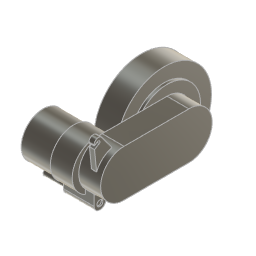
robotCad (Autodesk Fusion 360 archive; units mm, degrees)
design "silnikLewyDok"
Autodesk Fusion 360 part; units mm, degrees
sketch "Szkic1" plane through (0, 0, 0) normal (1, 0, 0) x (0, 1, 0)
  circle A0 centre (0, 0) radius 32.5
  dimension "d1" = 65
  constraint coincident A0.centre origin
  measures "d1" diameter of A0
extrude "Wyciągnięcie proste1" add sketch "Szkic1" along normal blind 15.5 makes body 1
sketch "Szkic2" plane through (15.5, 0, 0) normal (1, 0, 0) x (0, 1, 0)
  circle A0 centre (0, 0) radius 32.5
  circle A1 centre (0, 0) radius 23
  dimension "d4" = 46
  constraint coincident A0.centre A1.centre
  measures "d4" diameter of A1
extrude "Wyciągnięcie proste2" add sketch "Szkic2" along normal blind 2 contours A1 bodies 1
sketch "Szkic3" plane through (17.5, 0, 0) normal (1, 0, 0) x (0, 1, 0)
  circle A0 centre (0, 0) radius 23
  circle A1 centre (0, 0) radius 16
  circle A2 centre (-44.5, 0) radius 16
  line L0 (-44.5, 16) -> (0, 16)
  line L1 (-44.5, -16) -> (0, -16)
  dimension "d7" = 32
  dimension "d8" = 32
  dimension "d9" = 44.5
  constraint concentric A0 A1
  constraint tangent A2 L0
  constraint tangent A1 L0
  constraint coincident A2 L0.start
  constraint tangent A1 L1
  constraint coincident A2 L1.start
  constraint tangent A2 L1
  constraint coincident A1 L1.end
  constraint coincident A1 L0.end
  measures "d7" diameter of A1
  measures "d8" diameter of A2
  measures "d9" distance of A0.centre A2.centre
extrude "Wyciągnięcie proste3" add sketch "Szkic3" along normal blind 15 contours A0 A1 L0 L1 | A0 A2 L0 L1 | A2 | A1 picked at (-15.8747, 13.172) bodies 1
sketch "Szkic4" plane through (17.5, 0, 0) normal (-1, 0, 0) x (0, -1, 0)
  arc A0 (16.5227, -16) -> (16.5227, 16) centre (0, 0) ccw
  line L0 (16.5227, -16) -> (44.5, -16)
  arc A1 (44.5, -16) -> (44.5, 16) centre (44.5, 0) ccw
  line L1 (44.5, 16) -> (16.5227, 16)
  circle A2 centre (49, 0) radius 16
  arc A3 (0, 16) -> (0, -16) centre (0, 0) ccw
  circle A4 centre (49, 0) radius 15
  dimension "d12" = 32
  dimension "d13" = 49
  dimension "d14" = 30
  constraint concentric A2 A4
  measures "d12" diameter of A2
  measures "d13" distance of A2.centre A0.centre
  measures "d14" diameter of A4
extrude "Wyciągnięcie proste4" add sketch "Szkic4" along normal blind 15 contours A1 A2 A4 | A1 A2 A4 bodies 1
sketch "Szkic5" plane through (17.5, 0, 0) normal (-1, 0, 0) x (0, -1, 0)
  arc A0 (50.1944, 14.9524) -> (50.1944, -14.9524) centre (49, 0) ccw
  arc A1 (50.1944, -14.9524) -> (50.1944, 14.9524) centre (44.5, 0) ccw
  circle A2 centre (49, 0) radius 15
  circle A3 centre (49, 0) radius 15
  constraint concentric A0 A2
  constraint tangent A2 A3
extrude "Wyciągnięcie proste5" add sketch "Szkic5" along normal blind 36 bodies 1
ref_plane "Płaszczyzna konstrukcyjna1" through (23.5, -22.25, 0) normal (1, 0, 0) x (0, 1, 0)
sketch "Szkic6" plane through (23.5, -22.25, 0) normal (1, 0, 0) x (0, 1, 0)
  circle A0 centre (-29.75, -18.5) radius 2
  circle A1 centre (-29.75, -18.5) radius 4
  arc A2 (-22.25, 16) -> (-22.25, -16) centre (-22.25, 0) ccw
  arc A3 (22.25, -16) -> (22.25, 16) centre (22.25, 0) ccw
  point P0 (-16, -22.5)
  dimension "d20" = 4
  dimension "d21" = 8
  dimension "d22" = 22.5
  dimension "d23" = 4
  dimension "d24" = 52
  constraint concentric A0 A1
  measures "d20" diameter of A0
  measures "d21" diameter of A1
  measures "d22" vertical distance of P0 A2.centre
  measures "d23" vertical distance of A0.centre P0
  measures "d24" horizontal distance of A0.centre A3.centre
extrude "Wyciągnięcie proste6" add sketch "Szkic6" against normal blind 21 separate body contours A1 A2 picked at (-33.0386, -18.0016) makes body 2
sketch "Szkic8" plane through (23.5, 0, 0) normal (1, 0, 0) x (0, 1, 0)
  circle A0 centre (-52, -18.5) radius 2
  circle A1 centre (-52, -18.5) radius 2
  arc A2 (-50.962, -14.637) -> (-50.0549, -15.0048) centre (-52, -18.5) ccw
  arc A3 (-50.962, -14.637) -> (-50.0549, -15.0048) centre (-44.5, 0) ccw
  constraint concentric A0 A1
extrude "Wyciągnięcie proste7" add sketch "Szkic8" along normal blind -37 and the other way blind 1 contours A0 A1 bodies 2
sketch "Szkic9" plane through (23.5, 0, 0) normal (1, 0, 0) x (0, 1, 0)
  line L0 (-48.4419, -20.3275) -> (-46.1741, -15.9122)
  arc A0 (-44.5, 16) -> (-44.5, -16) centre (-44.5, 0) ccw
  line L1 (-56, -18.5) -> (-56, -11.1243)
  line L2 (-46.1741, -15.9122) -> (-56, -11.1243)
  arc A1 (-50.962, -14.637) -> (-50.0549, -15.0048) centre (-52, -18.5) ccw
  arc A2 (-50.962, -14.637) -> (-50.0549, -15.0048) centre (-44.5, 0) ccw
  circle A3 centre (-52, -18.5) radius 2
  constraint tangent L0 A1
  constraint coincident L0.start A1
  constraint coincident L1.start A1
  constraint coincident A0 L1.end
  constraint vertical L1
  constraint coincident A0 L0.end
extrude "Wyciągnięcie proste8" add sketch "Szkic9" against normal up to surface (21 mm away) contours L0 A0 A1 | A0 L2 A2 | A0 L1 A1 bodies 1 2
ref_plane "Płaszczyzna konstrukcyjna2" through (28.5, -22.25, 0) normal (1, 0, 0) x (0, 1, 0)
sketch "Szkic10" plane through (28.5, -22.25, 0) normal (1, 0, 0) x (0, 1, 0)
  circle A0 centre (-35.75, 23) radius 3
  line L0 (-38.75, -16) -> (-38.75, 26) construction
  line L1 (-38.75, 26) -> (-16.3036, 26) construction
  line L2 (-22.25, -16) -> (22.25, -16)
  arc A1 (-24.5, 15.841) -> (-33.75, -14.3875) centre (-26.75, 0) ccw
  arc A2 (-22.25, 16) -> (-22.25, -16) centre (-22.25, 0) ccw
  line L3 (-38.75, 23) -> (-37.0399, 6.104)
  line L4 (-33.5801, 25.0716) -> (-26.5025, 15.4245)
  dimension "d35" = 6
  dimension "d36" = 42
  dimension "d37" = 16.5
  constraint vertical L0
  constraint perpendicular L0 L1
  constraint tangent A0 L1
  constraint coincident L0.start L2
  constraint tangent A0 L0
  constraint coincident A0 L3.start
  constraint coincident A2 L3.end
  constraint coincident A0 L4.start
  constraint coincident A2 L4.end
  measures "d35" diameter of A0
  measures "d36" distance of L0.start L0.end
  measures "d37" distance of L0 A2.centre
extrude "Wyciągnięcie proste9" add sketch "Szkic10" against normal blind 3.5 contours A0 L3 L4 | A0 A1 L3 L4 | A1 A2 L3 L4 bodies 1
sketch "Szkic11" plane through (28.5, 0, 0) normal (1, 0, 0) x (0, 1, 0)
  line L0 (-61, 23) -> (-59.2899, 6.104)
  arc A0 (-48.7525, 15.4245) -> (-59.2899, 6.104) centre (-44.5, 0) ccw
  line L1 (-48.7525, 15.4245) -> (-55.8301, 25.0716)
  arc A1 (-55.8301, 25.0716) -> (-61, 23) centre (-58, 23) ccw
  circle A2 centre (-58, 23) radius 1
  line L2 (-57.4724, 22.1505) -> (-60.7105, 20.1395)
  line L3 (-58.4492, 23.8935) -> (-61.2557, 22.1505)
  dimension "d40" = 2
  constraint concentric A1 A2
  constraint coincident A2 L2.start
  constraint coincident L0 L2.end
  constraint tangent A2 L2
  constraint coincident A2 L3.start
  constraint parallel L2 L3
  measures "d40" distance of A1 A2
extrude "Wyciągnięcie proste10" cut sketch "Szkic11" against normal blind 10 contours A2 | L0 A2 L2 L3 bodies 1
equation "d9 = 75.5 mm - 31 mm"
equation "d13 = 81 mm - 32 mm"
equation "d22 = 38.5 mm - 16 mm"
equation "d24 = 56 mm - 4 mm"

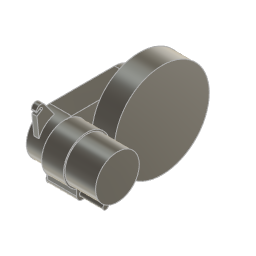
design "silnikPrawyDok"
Autodesk Fusion 360 part; units mm, degrees
sketch "Szkic1" plane through (0, 0, 0) normal (1, 0, 0) x (0, 1, 0)
  circle A0 centre (0, 0) radius 32.5
  dimension "d1" = 65
  constraint coincident A0.centre origin
  measures "d1" diameter of A0
extrude "Wyciągnięcie proste1" add sketch "Szkic1" along normal blind 15.5 makes body 1
sketch "Szkic2" plane through (0, 0, 0) normal (1, 0, 0) x (0, 1, 0)
  circle A0 centre (0, 0) radius 32.5
  circle A1 centre (0, 0) radius 23
  circle A2 centre (0, 0) radius 32.5
  dimension "d4" = 46
  constraint coincident A0.centre A1.centre
  measures "d4" diameter of A1
extrude "Wyciągnięcie proste2" add sketch "Szkic2" against normal blind 2 contours A1 bodies 1
sketch "Szkic3" plane through (-2, 0, 0) normal (-1, 0, 0) x (0, 1, 0)
  circle A0 centre (0, 0) radius 23
  circle A1 centre (0, 0) radius 16
  circle A2 centre (-44.5, 0) radius 16
  line L0 (-44.5, 16) -> (0, 16)
  line L1 (-44.5, -16) -> (0, -16)
  dimension "d7" = 32
  dimension "d8" = 32
  dimension "d9" = 44.5
  constraint concentric A0 A1
  constraint tangent A2 L0
  constraint tangent A1 L0
  constraint coincident A2 L0.start
  constraint tangent A1 L1
  constraint coincident A2 L1.start
  constraint tangent A2 L1
  constraint coincident A1 L1.end
  constraint coincident A1 L0.end
  measures "d7" diameter of A1
  measures "d8" diameter of A2
  measures "d9" distance of A0.centre A2.centre
extrude "Wyciągnięcie proste3" add sketch "Szkic3" along normal blind 15 contours A0 A1 L0 L1 | A0 A2 L0 L1 | A2 | A1 picked at (-15.8747, 13.172) bodies 1
sketch "Szkic4" plane through (-2, 0, 0) normal (1, 0, 0) x (0, -1, 0)
  arc A0 (16.5227, -16) -> (16.5227, 16) centre (0, 0) ccw
  line L0 (16.5227, -16) -> (44.5, -16)
  arc A1 (44.5, -16) -> (44.5, 16) centre (44.5, 0) ccw
  line L1 (44.5, 16) -> (16.5227, 16)
  circle A2 centre (49, 0) radius 16
  arc A3 (0, 16) -> (0, -16) centre (0, 0) ccw
  circle A4 centre (49, 0) radius 15
  dimension "d12" = 32
  dimension "d13" = 49
  dimension "d14" = 30
  constraint concentric A2 A4
  measures "d12" diameter of A2
  measures "d13" distance of A2.centre A0.centre
  measures "d14" diameter of A4
extrude "Wyciągnięcie proste4" add sketch "Szkic4" along normal blind 15 contours A1 A2 A4 | A1 A2 A4 bodies 1
sketch "Szkic5" plane through (-2, 0, 0) normal (1, 0, 0) x (0, -1, 0)
  arc A0 (50.1944, 14.9524) -> (50.1944, -14.9524) centre (49, 0) ccw
  arc A1 (50.1944, -14.9524) -> (50.1944, 14.9524) centre (44.5, 0) ccw
  circle A2 centre (49, 0) radius 15
  circle A3 centre (49, 0) radius 15
  constraint concentric A0 A2
  constraint tangent A2 A3
extrude "Wyciągnięcie proste5" add sketch "Szkic5" along normal blind 36 bodies 1
ref_plane "Płaszczyzna konstrukcyjna1" through (-8, -22.25, 0) normal (-1, 0, 0) x (0, 1, 0)
sketch "Szkic6" plane through (-8, -22.25, 0) normal (-1, 0, 0) x (0, 1, 0)
  circle A0 centre (-29.75, -18.5) radius 2
  circle A1 centre (-29.75, -18.5) radius 4
  arc A2 (-22.25, 16) -> (-22.25, -16) centre (-22.25, 0) ccw
  arc A3 (22.25, -16) -> (22.25, 16) centre (22.25, 0) ccw
  line L0 (42.25, 0) -> (24.75, 0)
  circle A4 centre (-29.75, 18.5) radius 2
  circle A5 centre (-29.75, 18.5) radius 4
  point P0 (-16, -22.5)
  dimension "d20" = 4
  dimension "d21" = 8
  dimension "d22" = 22.5
  dimension "d23" = 4
  dimension "d24" = 52
  constraint concentric A0 A1
  constraint symmetric A0 L0 A4
  constraint symmetric A1 L0 A5
  measures "d20" diameter of A0
  measures "d21" diameter of A1
  measures "d22" vertical distance of P0 A2.centre
  measures "d23" vertical distance of A0.centre P0
  measures "d24" horizontal distance of A0.centre A3.centre
extrude "Wyciągnięcie proste6" add sketch "Szkic6" against normal blind 21 separate body contours A2 A5 picked at (-33.0386, 18.0016) makes body 2
sketch "Szkic8" plane through (-8, 0, 0) normal (-1, 0, 0) x (0, 1, 0)
  circle A0 centre (-52, -18.5) radius 2
  arc A1 (-50.0549, 15.0048) -> (-50.962, 14.637) centre (-44.5, 0) ccw
  circle A2 centre (-52, 18.5) radius 2
  arc A3 (-50.0549, 15.0048) -> (-50.962, 14.637) centre (-52, 18.5) ccw
extrude "Wyciągnięcie proste7" add sketch "Szkic8" along normal blind -37 and the other way blind 1 contours A2 bodies 2
sketch "Szkic9" plane through (-7, 0, 0) normal (-1, 0, 0) x (0, 1, 0)
  line L0 (-48.4419, -20.3275) -> (-46.1741, -15.9122)
  arc A0 (-44.5, 16) -> (-44.5, -16) centre (-44.5, 0) ccw
  line L1 (-56, -18.5) -> (-56, -11.1243)
  line L2 (-46.1741, -15.9122) -> (-56, -11.1243)
  arc A1 (-50.0549, 15.0048) -> (-50.962, 14.637) centre (-44.5, 0) ccw
  circle A2 centre (-52, 18.5) radius 2
  circle A3 centre (-52, 18.5) radius 2
  arc A4 (-50.0549, 15.0048) -> (-50.962, 14.637) centre (-52, 18.5) ccw
  line L3 (20, 0) -> (2.5, 0)
  line L4 (-56, 18.5) -> (-56, 11.1243)
  line L5 (-46.1741, 15.9122) -> (-56, 11.1243)
  line L6 (-48.4419, 20.3275) -> (-46.1741, 15.9122)
  point P0 (-44.5, 16)
  constraint coincident A0 L1.end
  constraint vertical L1
  constraint coincident A0 L0.end
  constraint symmetric L0.start L3 L6.start
  constraint symmetric A0.end L3 P0
  constraint symmetric L0.end L3 L5.start
  constraint symmetric L1.start L3 L4.start
  constraint symmetric L1.end L3 L4.end
extrude "Wyciągnięcie proste8" add sketch "Szkic9" against normal up to surface (20 mm away) contours A0 A1 L5 | A0 A4 L6 | A0 A4 L4 bodies 1 2
ref_plane "Płaszczyzna konstrukcyjna2" through (-13, -22.25, 0) normal (-1, 0, 0) x (0, 1, 0)
sketch "Szkic10" plane through (-13, -22.25, 0) normal (-1, 0, 0) x (0, 1, 0)
  circle A0 centre (-35.75, 23) radius 3
  line L0 (-38.75, -16) -> (-38.75, 26) construction
  line L1 (-38.75, 26) -> (-16.3036, 26) construction
  line L2 (-22.25, -16) -> (22.25, -16)
  arc A1 (-33.75, 14.3875) -> (-24.5, -15.841) centre (-26.75, 0) ccw
  arc A2 (-22.25, 16) -> (-22.25, -16) centre (-22.25, 0) ccw
  line L3 (-38.75, 23) -> (-37.0399, 6.104)
  line L4 (-33.5801, 25.0716) -> (-26.5025, 15.4245)
  line L5 (42.25, 0) -> (24.75, 0)
  line L6 (-33.5801, -25.0716) -> (-26.5025, -15.4245)
  circle A3 centre (-35.75, -23) radius 3
  line L7 (-38.75, -23) -> (-37.0399, -6.104)
  point P0 (-22.25, -16)
  point P1 (-33.75, -14.3875)
  point P2 (-38.75, -26)
  dimension "d35" = 6
  dimension "d36" = 42
  dimension "d37" = 16.5
  constraint vertical L0
  constraint perpendicular L0 L1
  constraint tangent A0 L1
  constraint coincident L0.start L2
  constraint tangent A0 L0
  constraint coincident A0 L3.start
  constraint coincident A2 L3.end
  constraint coincident A0 L4.start
  constraint coincident A2 L4.end
  constraint symmetric A0 L5 A3
  constraint symmetric L0.end L5 P2
  constraint symmetric A1.start L5 P1
  constraint symmetric A2.start L5 P0
  constraint symmetric L3.start L5 L7.start
  constraint symmetric L3.end L5 L7.end
  constraint symmetric L4.start L5 L6.start
  constraint symmetric L4.end L5 L6.end
  measures "d35" diameter of A0
  measures "d36" distance of L0.start L0.end
  measures "d37" distance of L0 A2.centre
extrude "Wyciągnięcie proste9" add sketch "Szkic10" against normal blind 3.5 contours A1 A2 L6 L7 | A1 L6 A3 L7 | L6 A3 L7 bodies 1
sketch "Szkic11" plane through (-13, 0, 0) normal (-1, 0, 0) x (0, 1, 0)
  arc A0 (-59.2899, -6.104) -> (-48.7525, -15.4245) centre (-44.5, 0) ccw
  circle A1 centre (-58, 23) radius 1
  line L0 (-57.4724, 22.1505) -> (-60.7105, 20.1395)
  line L1 (-58.4492, 23.8935) -> (-61.2557, 22.1505)
  line L2 (-55.8301, -25.0716) -> (-48.7525, -15.4245)
  line L3 (-59.2899, -6.104) -> (-61, -23)
  arc A2 (-61, -23) -> (-55.8301, -25.0716) centre (-58, -23) ccw
  line L4 (20, 0) -> (2.5, 0)
  circle A3 centre (-58, -23) radius 1
  line L5 (-57.4724, -22.1505) -> (-60.7105, -20.1395)
  line L6 (-58.4492, -23.8935) -> (-61.2557, -22.1505)
  constraint coincident A1 L0.start
  constraint tangent A1 L0
  constraint coincident A1 L1.start
  constraint parallel L0 L1
  constraint symmetric A1 L4 A3
  constraint symmetric L0.start L4 L5.start
  constraint symmetric L0.end L4 L5.end
  constraint symmetric L1.start L4 L6.start
  constraint symmetric L1.end L4 L6.end
extrude "Wyciągnięcie proste10" cut sketch "Szkic11" against normal blind 10 contours L3 A3 L5 L6 | A3 L6 | A1 L1 picked at (-57.7688, -22.7789) picked at (-57.8523, 23.2601) bodies 1
equation "d9 = 75.5 mm - 31 mm"
equation "d13 = 81 mm - 32 mm"
equation "d22 = 38.5 mm - 16 mm"
equation "d24 = 56 mm - 4 mm"

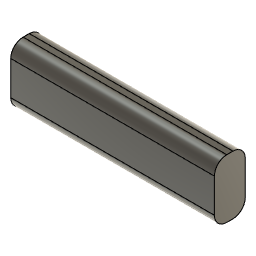
design "bat4s1p_dluga"
Autodesk Fusion 360 part; units mm, degrees
sketch "Szkic1" plane through (0, 0, 0) normal (1, 0, 0) x (0, 1, 0)
  line L0 (8, 25) -> (12, 25)
  line L1 (20, 17) -> (20, -5)
  line L2 (12, -13) -> (8, -13)
  line L3 (0, -5) -> (0, 17)
  arc A0 (8, 25) -> (0, 17) centre (8, 17) ccw
  arc A1 (20, 17) -> (12, 25) centre (12, 17) ccw
  arc A2 (12, -13) -> (20, -5) centre (12, -5) ccw
  arc A3 (0, -5) -> (8, -13) centre (8, -5) ccw
  point P0 (0, 25)
  point P1 (20, 25)
  point P2 (20, -13)
  dimension "d1" = 20
  dimension "d2" = 38
  dimension "d3" = 8
  dimension "d4" = 8
  constraint horizontal L0
  constraint vertical L1
  constraint horizontal L2
  constraint vertical L3
  constraint coincident P0 L0
  constraint coincident P0 L3
  constraint tangent L0 A0
  constraint tangent L3 A0
  constraint coincident P1 L0
  constraint coincident P1 L1
  constraint tangent L0 A1
  constraint tangent L1 A1
  constraint coincident P2 L1
  constraint coincident P2 L2
  constraint tangent L1 A2
  constraint tangent L2 A2
  constraint equal A1 A2
  constraint tangent L2 A3
  constraint tangent L3 A3
  constraint equal A1 A3
  measures "d1" distance of P0 P1
  measures "d2" distance of P1 P2
  measures "d3" radius of A0
  measures "d4" radius of A1
extrude "Wyciągnięcie proste1" add sketch "Szkic1" along normal blind 132
